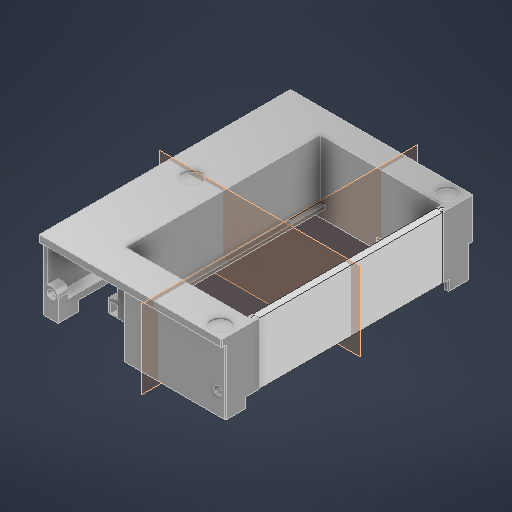
# Autodesk Inventor part: Kameraturm_Base_V3
Saved by Autodesk Inventor 2026.1 (Build 301233020, 233B)
## iProperties
Created: 2025-08-17
Part Number: Kameraturm_Base_V3
Material: Generic
Document SubType Name: Modeling
Designer: peter
Density: 1 g/cm^3
Appearance: Default
Author: peter
Autodesk Inventor part; units mm, degrees
sketch "Sketch1" plane through (0, 0, 0) normal (0, 0, 1) x (1, 0, 0)
  line L0 (135, 183) -> (0, 183) projected
  line L1 (0, 180) -> (0, 183) projected
  line L2 (0, 180) -> (135, 180) projected
  line L3 (135, 180) -> (135, 183) projected
  line L4 (0, -3) -> (135, -3) projected
  line L5 (135, 0) -> (135, -3) projected
  line L6 (135, 0) -> (0, 0) projected
  line L7 (0, 0) -> (0, -3) projected
  line L8 (0, 183) -> (135, 183)
  line L9 (135, 183) -> (135, -3)
  line L10 (135, -3) -> (0, -3)
  line L11 (0, -3) -> (0, 183)
  point P0 (135, 180)
  constraints: 8 end point, 2 parallel, 1 horizontal, 1 perpendicular
extrude "Extrusion1" add sketch "Sketch1" against normal blind 40 contours L9 L6 L11 L2
sketch "Sketch2" plane through (0, 0, 0) normal (0, 0, 1) x (1, 0, 0)
  line L0 (135, 180) -> (135, 0) construction
  line L1 (135, 90) -> (0, 90) construction
  line L2 (0, 0) -> (0, 180) construction
  line L3 (40, 165) -> (130, 165)
  line L4 (130, 165) -> (130, 15)
  line L5 (130, 15) -> (40, 15)
  line L6 (40, 15) -> (40, 165)
  line L7 (40, 165) -> (130, 15) construction
  line L8 (130, 165) -> (40, 15) construction
  line L9 (40, 15) -> (130, 15)
  line L10 (130, 15) -> (130, 21)
  line L11 (130, 21) -> (40, 21)
  line L12 (40, 21) -> (40, 15)
  point P0 (85, 90)
  dimension "d2" = 90
  dimension "d3" = 150
  dimension "d4" = 5
  dimension "d67" = 6
  constraints: 22 end point, 4 midpoint, 4 parallel, 2 horizontal, 2 perpendicular, 2 point on line
  measures "d2" distance of L4.end L5.end
  measures "d3" distance of L3.end L4.end
  measures "d4" distance between parallel lines of L0 L4
  measures "d67" distance of L10.end L9.end
extrude "Extrusion2" cut sketch "Sketch2" against normal through all contours L3 L4 L11 L6
sketch "Sketch3" plane through (0, 0, 0) normal (0, 0, 1) x (1, 0, 0)
  line L0 (135, 0) -> (0, 0) projected
  line L1 (60, 0) -> (3, 0)
  line L2 (3, 0) -> (3, 18)
  line L3 (3, 18) -> (60, 18)
  line L4 (60, 18) -> (60, 0)
  line L5 (3, 18) -> (37, 18)
  line L6 (37, 18) -> (37, 40.7573)
  line L7 (37, 40.7573) -> (3, 40.7573)
  line L8 (3, 40.7573) -> (3, 18)
  line L9 (40, 21) -> (40, 165) projected
  line L10 (0, 180) -> (0, 0) projected
  line L11 (130, 21) -> (40, 21) projected
  point P0 (37, 18)
  dimension "d8" = 3
  dimension "d9" = 3
  dimension "d10" = 60
  dimension "d68" = 3
  constraints: 16 end point, 4 parallel, 2 horizontal, 2 perpendicular, 1 point on line
  measures "d8" distance between parallel lines of L9 L6
  measures "d9" distance between parallel lines of L10 L8
  measures "d10" distance between parallel lines of L10 L4
  measures "d68" distance between parallel lines of L11 L3
extrude "Extrusion3" cut sketch "Sketch3" against normal blind 36
ref_plane "Work Plane1" through (-62, 12.5, -48) normal (0, 0, 1) x (1, 0, 0)
sketch "Sketch4" plane through (0, 0, -40) normal (0, 0, -1) x (-1, 0, 0)
  line L0 (0, -2.5) -> (0, 22) projected
  line L1 (0, 158) -> (0, 182.5) projected
  line L2 (125, -2.5) -> (125, 182.5) projected
  line L3 (-478, 162.5) -> (92, 162.5) projected
  line L4 (92, 17.5) -> (-478, 17.5) projected
  line L5 (-135, 180) -> (-135, 0) projected
  line L6 (0, 0) -> (-135, 0)
  line L7 (-135, 0) -> (-135, 15)
  line L8 (-135, 15) -> (0, 15)
  line L9 (0, 15) -> (0, 0)
  line L10 (0, 180) -> (-135, 180) projected
  line L11 (0, 180) -> (-135, 180)
  line L12 (-135, 180) -> (-135, 165)
  line L13 (-135, 165) -> (0, 165)
  line L14 (0, 165) -> (0, 180)
  line L15 (125, 182.5) -> (0, 182.5) projected
  line L16 (0, -2.5) -> (125, -2.5) projected
  line L17 (100, 22) -> (0, 22) projected
  line L18 (100, 22) -> (100, 158) projected
  line L19 (0, 158) -> (100, 158) projected
  circle A0 centre (80, 170.25) radius 7.05 projected
  circle A1 centre (40, 170.25) radius 7.05 projected
  point P0 (100, 22.5)
  point P1 (100, 157.5)
  point P2 (-130, 15)
  point P3 (-130, 165)
  constraints: 16 end point, 4 parallel, 2 horizontal, 2 horizontal alignment, 2 perpendicular, 2 point on line
extrude "Extrusion4" add sketch "Sketch4" along normal up to surface (8 mm away) contours L6 L5 L8 L0 | L1 L13 L5 L10
sketch "Sketch5" plane through (0, 180, 0) normal (0, 1, 0) x (1, 0, 0)
  line L0 (135, 25) -> (0, 25) projected
  line L1 (60, 0) -> (135, 0) projected
  line L2 (135, 0) -> (0, 0)
  line L3 (0, 0) -> (0, 25)
  line L4 (0, 25) -> (135, 25)
  line L5 (135, 25) -> (135, 0)
  point P0 (0, 0)
  constraints: 8 end point, 2 parallel, 1 horizontal, 1 perpendicular
ref_plane "Work Plane2" through (-120, 183, -97.3) normal (0, 1, 0) x (0, 0, 1)
extrude "Extrusion5" add sketch "Sketch5" along normal up to surface (3 mm away)
sketch "Sketch8" plane through (0, 0, 0) normal (0, 0, 1) x (1, 0, 0)
  line L0 (670, 183) -> (135, 183) projected
  line L1 (0, -3) -> (135, -3) projected
  line L2 (135, 183) -> (0, 183)
  line L3 (0, 183) -> (0, -3)
  line L4 (0, -3) -> (135, -3)
  line L5 (135, -3) -> (135, 183)
  line L6 (3, 0) -> (3, 40.7573) projected
  line L7 (3, 40.7573) -> (37, 40.7573) projected
  line L8 (37, 40.7573) -> (37, 18) projected
  line L9 (37, 18) -> (60, 18) projected
  line L10 (60, 18) -> (60, 0) projected
  line L11 (60, 0) -> (135, 0) projected
  line L12 (135, 0) -> (135, 183) projected
  line L13 (135, 183) -> (0, 183) projected
  line L14 (0, 183) -> (0, 0) projected
  line L15 (0, 0) -> (3, 0) projected
  line L16 (130, 165) -> (130, 21) projected
  line L17 (40, 21) -> (40, 165) projected
  line L18 (40, 165) -> (130, 165) projected
  line L19 (60, 0) -> (0, 0)
  line L20 (130, 21) -> (40, 21) projected
  constraints: 10 end point, 3 parallel, 1 horizontal, 1 perpendicular
extrude "Extrusion8" add sketch "Sketch8" along normal blind 5
sketch "Sketch9" plane through (0, 0, 5) normal (0, 0, 1) x (1, 0, 0)
  circle A0 centre (125, 174) radius 7.05
  circle A1 centre (125, 6) radius 7.05
  line L0 (135, -3) -> (135, 183) projected
  line L1 (135, 183) -> (0, 183) projected
  line L2 (0, -3) -> (135, -3) projected
  line L3 (0, 183) -> (0, -3) projected
  circle A2 centre (20, 90) radius 7.05
  line L4 (0, 90) -> (40, 90) construction
  line L5 (40, 165) -> (40, 21) projected
  point P0 (0, 0)
  point P1 (40, 15)
  dimension "d31" = 14.1
  dimension "d35" = 10
  dimension "d36" = 9
  dimension "d37" = 9
  constraints: 3 centre point, 3 midpoint, 2 end point, 2 equal radius, 1 coincident, 1 horizontal alignment, 1 point on line, 1 vertical alignment
  measures "d31" diameter of A0
  measures "d35" distance from line of L0 A0.centre
  measures "d36" distance from line of L1 A0.centre
  measures "d37" distance from line of L2 A1.centre
extrude "Extrusion9" cut sketch "Sketch9" against normal blind 1.5 contours A0 | A1 | A2
chamfer "Chamfer1" distance 0.5 angle 45 14 edges at (135, 183, 2.5) (135, 183, -12.5) (0, 183, -12.5) (0, 183, 2.5) (0, 0, -24) (135, 0, -24) (135, -3, 2.5) (0, -3, 2.5) (135, 180, -36.5) (0, 180, -36.5) (135, 15, -44) (135, 165, -44) (0, 15, -44) (0, 165, -44)
ref_plane "Work Plane3" through (0, 0, 0) normal (0, 0, 1) x (1, 0, 0)
ref_plane "Work Plane4" through (0, 0, -3) normal (0, 0, -1) x (-1, 0, 0)
sketch "Sketch12" plane through (0.5, 180, -25) normal (0, 1, 0) x (1, 0, 0)
  arc A0 (107.5, 4.5) -> (107.5, 9.5) centre (107.5, 7) ccw projected
  arc A1 (106.5, 9.5) -> (106.5, 4.5) centre (106.5, 7) ccw projected
  arc A2 (26.5, 9.5) -> (26.5, 4.5) centre (26.5, 7) ccw projected
  arc A3 (27.5, 4.5) -> (27.5, 9.5) centre (27.5, 7) ccw projected
  line L0 (107.5, 7) -> (106.5, 7)
  line L1 (27.5, 7) -> (26.5, 7)
  circle A4 centre (107, 7) radius 3.2
  circle A5 centre (27, 7) radius 3.2
  point P0 (-0.5, -25)
  dimension "d53" = 6.4
  dimension "d54" = 6.4
  constraints: 4 end point, 2 centre point, 2 horizontal, 2 midpoint
  measures "d53" diameter of A4
  measures "d54" diameter of A5
extrude "Extrusion12" cut sketch "Sketch12" against normal blind 12
sketch "Sketch13" plane through (3, 0, -36) normal (0, -1, 0) x (1, 0, 0)
  circle A0 centre (3, 4) radius 2.5 projected
  circle A1 centre (3, 4) radius 5
  line L0 (57, 0) -> (0, 0) projected
  line L1 (0, 0) -> (0, 36) projected
  line L2 (8, 4) -> (8, 0)
  line L3 (3, 9) -> (0, 9)
  circle A2 centre (3, 4) radius 3.2
  point P0 (-3, 36)
  dimension "d57" = 10
  dimension "d58" = 6.4
  constraints: 4 end point, 2 centre point, 2 coincident, 2 perpendicular, 2 point on circle, 2 point on line, 2 tangent
  measures "d57" diameter of A1
  measures "d58" diameter of A2
extrude "Extrusion13" add sketch "Sketch13" against normal blind 8 contours A1 L0 L1 A2 | L2 L0 A1 | A1 L1 L3 | A2 L1 picked at (0.1667, 4)
sketch "Sketch14" plane through (60, 0, -36) normal (0, -1, 0) x (1, 0, 0)
  circle A0 centre (-54, 4) radius 2.5 projected
  circle A1 centre (69, 4) radius 2.5 projected
  circle A2 centre (-54, 4) radius 3.2
  circle A3 centre (69, 4) radius 3.2
  point P0 (-60, 36)
  dimension "d61" = 6.4
  dimension "d62" = 6.4
  constraints: 2 centre point, 2 coincident
  measures "d61" diameter of A2
  measures "d62" diameter of A3
extrude "Extrusion14" cut sketch "Sketch14" against normal blind 12 contours A0 | A1 | A2 | A3
sketch "Sketch15" plane through (0, 0, -36) normal (0, 0, 1) x (1, 0, 0)
  line L0 (11, 8) -> (11, 0) projected
  line L1 (60, 0) -> (11, 0) projected
  line L2 (60, 18) -> (60, 0) projected
  line L3 (37, 18) -> (60, 18) projected
  line L4 (37, 40.7573) -> (37, 18) projected
  line L5 (3, 40.7573) -> (37, 40.7573) projected
  line L6 (3, 8) -> (3, 40.7573) projected
  line L7 (3, 8) -> (11, 8) projected
  line L8 (11, 0) -> (60, 0)
  line L9 (60, 0) -> (60, 18)
  line L10 (60, 18) -> (11, 18)
  line L11 (11, 18) -> (11, 0)
  line L12 (11, 18) -> (37, 18)
  line L13 (37, 18) -> (37, 40.7573)
  line L14 (37, 40.7573) -> (11, 40.7573)
  line L15 (11, 40.7573) -> (11, 18)
  point P0 (0, 0)
  constraints: 16 end point, 4 parallel, 2 horizontal, 2 perpendicular
extrude "Extrusion15" cut sketch "Sketch15" against normal through all contours L11 L10 L3 L2 L1 L0 | L15 L5 L4 L10
ref_plane "Work Plane5" through (0, 0, -40) normal (0, 0, -1) x (-1, 0, 0)
sketch "Sketch16" plane through (0, 0, -40) normal (0, 0, -1) x (-1, 0, 0)
  line L0 (-11, 40.7573) -> (-11, 15) projected
  line L1 (-11, 15) -> (-0.5, 15) projected
  line L2 (0, 14.5) -> (-0.5, 15) projected
  line L3 (0, 14.5) -> (0, 165.5) projected
  line L4 (-0.5, 165) -> (0, 165.5) projected
  line L5 (-0.5, 165) -> (-40, 165) projected
  line L6 (-40, 165) -> (-40, 21) projected
  line L7 (-40, 21) -> (-130, 21) projected
  line L8 (-130, 21) -> (-130, 165) projected
  line L9 (-130, 165) -> (-134.5, 165) projected
  line L10 (-135, 165.5) -> (-134.5, 165) projected
  line L11 (-135, 165.5) -> (-135, 14.5) projected
  line L12 (-134.5, 15) -> (-135, 14.5) projected
  line L13 (-134.5, 15) -> (-60, 15) projected
  line L14 (-60, 15) -> (-60, 18) projected
  line L15 (-60, 18) -> (-37, 18) projected
  line L16 (-37, 18) -> (-37, 40.7573) projected
  line L17 (-37, 40.7573) -> (-11, 40.7573) projected
  line L18 (-40, 21) -> (-130, 21)
  line L19 (-130, 21) -> (-130, 24)
  line L20 (-130, 24) -> (-40, 24)
  line L21 (-40, 24) -> (-40, 21)
  line L22 (-40, 21) -> (-43, 21)
  line L23 (-43, 21) -> (-43, 41)
  line L24 (-43, 41) -> (-40, 41)
  line L25 (-40, 41) -> (-40, 21)
  line L26 (-40, 41) -> (-43, 41)
  line L27 (-43, 41) -> (-43, 141)
  line L28 (-43, 141) -> (-40, 141)
  line L29 (-40, 141) -> (-40, 41)
  line L30 (-134.5, 165) -> (-0.5, 165) projected
  line L31 (-40, 141) -> (-43, 141)
  line L32 (-43, 141) -> (-43, 165)
  line L33 (-43, 165) -> (-40, 165)
  line L34 (-40, 165) -> (-40, 141)
  point P0 (0, 0)
  point P1 (-43, 24)
  point P2 (-43, 41)
  dimension "d72" = 3
  dimension "d73" = 3
  dimension "d74" = 20
  dimension "d75" = 3
  dimension "d76" = 100
  dimension "d77" = 3
  constraints: 32 end point, 8 parallel, 4 horizontal, 4 perpendicular, 1 point on line, 1 vertical alignment
  measures "d72" distance of L18.end L19.end
  measures "d73" distance of L23.end L24.end
  measures "d74" distance of L22.end L23.end
  measures "d75" distance of L27.end L28.end
  measures "d76" distance of L26.end L27.end
  measures "d77" distance of L32.end L33.end
extrude "Extrusion16" add sketch "Sketch16" against normal blind 2 separate body contours L6 L28 L32 L30 | L6 L20 L23 L24 | L6 L7 L23 L20 | L20 L23 L7 L8
extrude "Extrusion17" add sketch "Sketch16" against normal blind 2 contours L17 L16 L15 L14 L13 L12 L11 L10 L9 L8 L7 L6 L5 L4 L3 L2 L1 L0 | L6 L24 L27 L28 bodies 1
sketch "Sketch17" plane through (0, 0, -40) normal (0, 0, -1) x (-1, 0, 0)
  line L0 (-134.5, 165) -> (-135, 165.5) construction
  line L1 (-135, 14.5) -> (-135, 165.5) construction
  line L2 (-135, 0.5) -> (-135, 14.5) construction
  line L3 (-134.5, 0) -> (-135, 0.5) construction
  line L4 (-60, 0) -> (-134.5, 0) construction
  line L5 (-60, 15) -> (-60, 0) construction
  line L6 (-134.5, 15) -> (-60, 15) construction
  line L7 (-135, 14.5) -> (-134.5, 15) construction
  line L8 (-130, 165) -> (-134.5, 165) construction
  line L9 (-130, 165) -> (-130, 21) construction
  line L10 (-130, 21) -> (-40, 21) construction
  line L11 (-40, 21) -> (-40, 41) construction
  line L12 (-40, 41) -> (-43, 41) construction
  line L13 (-43, 41) -> (-43, 141) construction
  line L14 (-43, 141) -> (-40, 141) construction
  line L15 (-40, 141) -> (-40, 165) construction
  line L16 (-0.5, 165) -> (-40, 165) construction
  line L17 (0, 165.5) -> (-0.5, 165) construction
  line L18 (0, 179.5) -> (0, 165.5) construction
  line L19 (-0.5, 180) -> (0, 179.5) construction
  line L20 (-134.5, 180) -> (-0.5, 180) construction
  line L21 (-135, 179.5) -> (-134.5, 180) construction
  line L22 (-135, 165.5) -> (-135, 179.5) construction
  line L23 (-60, 18) -> (-60, 15) construction
  line L24 (-37, 18) -> (-60, 18) construction
  line L25 (-37, 40.7573) -> (-37, 18) construction
  line L26 (-11, 40.7573) -> (-37, 40.7573) construction
  line L27 (-11, 15) -> (-11, 40.7573) construction
  line L28 (-11, 0) -> (-11, 15) construction
  line L29 (-0.5, 0) -> (-11, 0) construction
  line L30 (0, 0.5) -> (-0.5, 0) construction
  line L31 (0, 14.5) -> (0, 0.5) construction
  line L32 (0, 165.5) -> (0, 14.5) construction
  line L33 (-40, 165) -> (-130, 165) construction
  line L34 (-11, 15) -> (-0.5, 15) construction
  line L35 (-0.5, 15) -> (0, 14.5) construction
  line L36 (-40, 165) -> (-40, 141) construction
  line L37 (-40, 141) -> (-43, 141) construction
  line L38 (-43, 141) -> (-43, 165) construction
  line L39 (-43, 165) -> (-40, 165) construction
  line L40 (-130, 24) -> (-43, 24) construction
  line L41 (-43, 24) -> (-43, 41) construction
  line L42 (-43, 41) -> (-40, 41) construction
  line L43 (-40, 41) -> (-40, 21) construction
  line L44 (-40, 21) -> (-130, 21) construction
  line L45 (-130, 21) -> (-130, 24) construction
  line L46 (-130, 24) -> (-43, 24)
  line L47 (-43, 24) -> (-43, 165)
  line L48 (-43, 165) -> (-130, 165)
  line L49 (-130, 165) -> (-130, 24)
  line L50 (-130, 25) -> (-44, 25)
  line L51 (-44, 25) -> (-44, 165)
  line L52 (-44, 165) -> (-130, 165)
  line L53 (-130, 165) -> (-130, 25)
  point P0 (0, 0)
  dimension "d82" = 1
  dimension "d83" = 1
  constraints: 16 end point, 4 parallel, 2 horizontal, 2 perpendicular, 2 point on line
  measures "d82" distance between parallel lines of L13 L51
  measures "d83" distance between parallel lines of L50 L40
extrude "Extrusion18" add sketch "Sketch17" against normal blind 2 contours L49 L50 L51 L48 L47 L46 bodies 1
sketch "Sketch18" plane through (0, 0, -40) normal (0, 0, -1) x (-1, 0, 0)
  line L0 (-43, 41) -> (-43, 24) projected
  line L1 (-43, 24) -> (-130, 24) projected
  line L2 (-130, 24) -> (-130, 21) projected
  line L3 (-130, 21) -> (-40, 21) projected
  line L4 (-40, 21) -> (-40, 41) projected
  line L5 (-40, 41) -> (-43, 41) projected
  line L6 (-134.5, 165) -> (-135, 165.5) projected
  line L7 (-135, 14.5) -> (-135, 165.5) projected
  line L8 (-135, 0.5) -> (-135, 14.5) projected
  line L9 (-134.5, 0) -> (-135, 0.5) projected
  line L10 (-60, 0) -> (-134.5, 0) projected
  line L11 (-60, 15) -> (-60, 0) projected
  line L12 (-134.5, 15) -> (-60, 15) projected
  line L13 (-135, 14.5) -> (-134.5, 15) projected
  line L14 (-130, 165) -> (-134.5, 165) projected
  line L15 (-130, 165) -> (-130, 25) projected
  line L16 (-130, 25) -> (-44, 25) projected
  line L17 (-44, 25) -> (-44, 165) projected
  line L18 (-43, 165) -> (-44, 165) projected
  line L19 (-43, 165) -> (-43, 141) projected
  line L20 (-43, 141) -> (-40, 141) projected
  line L21 (-40, 141) -> (-40, 165) projected
  line L22 (-0.5, 165) -> (-40, 165) projected
  line L23 (0, 165.5) -> (-0.5, 165) projected
  line L24 (0, 179.5) -> (0, 165.5) projected
  line L25 (-0.5, 180) -> (0, 179.5) projected
  line L26 (-134.5, 180) -> (-0.5, 180) projected
  line L27 (-135, 179.5) -> (-134.5, 180) projected
  line L28 (-135, 165.5) -> (-135, 179.5) projected
  line L29 (-60, 18) -> (-60, 15) projected
  line L30 (-37, 18) -> (-60, 18) projected
  line L31 (-37, 40.7573) -> (-37, 18) projected
  line L32 (-11, 40.7573) -> (-37, 40.7573) projected
  line L33 (-11, 15) -> (-11, 40.7573) projected
  line L34 (-11, 15) -> (-0.5, 15) projected
  line L35 (-0.5, 15) -> (0, 14.5) projected
  line L36 (0, 165.5) -> (0, 14.5) projected
  line L37 (-44, 165) -> (-130, 165) projected
  line L38 (-40, 165) -> (-43, 165) projected
  line L39 (-11, 0) -> (-11, 15) projected
  line L40 (-0.5, 0) -> (-11, 0) projected
  line L41 (0, 0.5) -> (-0.5, 0) projected
  line L42 (0, 14.5) -> (0, 0.5) projected
  line L43 (-40, 165) -> (-40, 141) projected
  line L44 (-40, 141) -> (-43, 141) projected
  line L45 (-43, 141) -> (-43, 165) projected
  line L46 (-43, 165) -> (-40, 165) projected
  line L47 (-130, 24) -> (-43, 24) projected
  line L48 (-43, 24) -> (-43, 41) projected
  line L49 (-43, 41) -> (-40, 41) projected
  line L50 (-40, 41) -> (-40, 21) projected
  line L51 (-40, 21) -> (-130, 21) projected
  line L52 (-130, 21) -> (-130, 24) projected
  point P0 (0, 0)
extrude "Extrusion19" add sketch "Sketch18" along normal blind 0.6 contours L5 L4 L3 L2 L1 L0 | L14 L15 L16 L17 L18 L19 L20 L21 L22 L23 L36 L35 L34 L33 L32 L31 L30 L29 L12 L13 L7 L6 | L38 L21 L20 L19 bodies 1
sketch "Sketch19" plane through (60, 0, -48) normal (0, 0, -1) x (-1, 0, 0)
  line L0 (0, 15) -> (-74.5, 15) projected
  line L1 (-22, 15) -> (-72, 15)
  line L2 (-72, 15) -> (-72, 2)
  line L3 (-72, 2) -> (-22, 2)
  line L4 (-22, 2) -> (-22, 15)
  line L5 (16, 165) -> (16, 25) projected
  line L6 (-74.5, 165) -> (59.5, 165) projected
  line L7 (-72, 165) -> (-22, 165)
  line L8 (-22, 165) -> (-22, 178)
  line L9 (-22, 178) -> (-72, 178)
  line L10 (-72, 178) -> (-72, 165)
  point P0 (60, 0)
  dimension "d89" = 38
  dimension "d92" = 50
  dimension "d93" = 13
  dimension "d94" = 13
  constraints: 16 end point, 5 parallel, 2 horizontal, 2 perpendicular, 2 point on line, 1 vertical alignment
  measures "d89" distance from line of L5 L1.start
  measures "d92" distance of L2.end L3.end
  measures "d93" distance of L3.end L1.start
  measures "d94" distance between parallel lines of L6 L9
extrude "Extrusion20" cut sketch "Sketch19" against normal blind 8.5 bodies 1
sketch "Sketch20" plane through (60, 0, -39.5) normal (0, 0, -1) x (-1, 0, 0)
  line L0 (-4.8389, 5.5) -> (-96.0854, 5.5) construction
  line L1 (-4.8389, 174.5) -> (-96.0854, 174.5) construction
  line L2 (-22, 2) -> (-72, 2) construction
  line L3 (-72, 178) -> (-22, 178) construction
  point P0 (60, 0)
  point P1 (-26.5, 5.5)
  point P2 (-42, 5.5)
  point P3 (-57.5, 5.5)
  point P4 (-47, 2)
  point P5 (-57.5, 174.5)
  point P6 (-42, 174.5)
  point P7 (-26.5, 174.5)
  point P8 (-47, 2)
  dimension "d97" = 3.5
  dimension "d98" = 3.5
  dimension "d99" = 15.5
  dimension "d100" = 15.5
  dimension "d149" = 5
  constraints: 6 point on line, 4 end point, 3 vertical alignment, 2 horizontal, 2 midpoint
  measures "d97" distance between parallel lines of L2 L0
  measures "d98" distance between parallel lines of L3 L1
  measures "d99" distance of point (-42, 5.5) point (-26.5, 5.5)
  measures "d100" distance of point (-42, 5.5) point (-57.5, 5.5)
  measures "d149" horizontal distance of point (-47, 2) point (-42, 5.5)
hole "Hole1" at (102, 5.5, -39.5) at (117.5, 5.5, -39.5) at (117.5, 174.5, -39.5) at (102, 174.5, -39.5) direction (0, 0, 1) diameter 4 depth 6 bodies 1
sketch "Sketch21" plane through (82, 2, -48) normal (1, 0, 0) x (0, 0, -1)
  circle A0 centre (-3.7, 6.5) radius 2.5
  line L0 (-7.4, 13) -> (0, 13) projected
  line L1 (0, 13) -> (0, 0) projected
  line L2 (-1.2, 9) -> (-6.2, 9)
  line L3 (-6.2, 9) -> (-6.2, 4)
  line L4 (-6.2, 4) -> (-1.2, 4)
  line L5 (-1.2, 4) -> (-1.2, 9)
  line L6 (-1.2, 9) -> (-6.2, 4) construction
  line L7 (-6.2, 9) -> (-1.2, 4) construction
  point P0 (-48, -2)
  point P1 (-3.7, 13)
  point P2 (0, 6.5)
  point P3 (-1.2, 6.5)
  point P4 (-3.7, 4)
  point P5 (-3.7, 9)
  point P6 (-6.2, 6.5)
  dimension "d112" = 5
  dimension "d147" = 5
  dimension "d148" = 5
  constraints: 12 end point, 4 midpoint, 2 parallel, 1 centre point, 1 horizontal, 1 horizontal alignment, 1 perpendicular, 1 vertical alignment
  measures "d112" diameter of A0
  measures "d147" distance of L4.end L3.end
  measures "d148" distance of L3.end L2.end
extrude "Extrusion22" cut sketch "Sketch21" against normal blind 30.75 bodies 1
sketch "Sketch22" plane through (0, 0, -40.6) normal (0, 0, -1) x (-1, 0, 0)
  line L0 (-37, 40.7573) -> (-11, 40.7573) projected
  line L1 (-82, 165) -> (-0.5, 165) projected
  line L2 (-32, 40.7573) -> (-37, 40.7573)
  line L3 (-37, 40.7573) -> (-37, 165)
  line L4 (-37, 165) -> (-32, 165)
  line L5 (-32, 165) -> (-32, 40.7573)
  line L6 (-44, 165) -> (-44, 25) projected
  line L7 (-32, 165) -> (-37, 165)
  line L8 (-37, 165) -> (-37, 173)
  line L9 (-37, 173) -> (-32, 173)
  line L10 (-32, 173) -> (-32, 165)
  line L11 (-40, 21) -> (-40, 165) projected
  point P0 (0, 0)
  dimension "d115" = 5
  dimension "d119" = 5
  dimension "d120" = 8
  dimension "d121" = 3
  constraints: 16 end point, 4 parallel, 2 horizontal, 2 perpendicular, 2 point on line
  measures "d115" distance of L3.end L4.end
  measures "d119" distance of L8.end L9.end
  measures "d120" distance of L7.end L8.end
  measures "d121" distance between parallel lines of L3 L11
extrude "Extrusion23" cut sketch "Sketch22" against normal blind 8 bodies 1
sketch "Sketch23" plane through (32, 173, -40.6) normal (0, -1, 0) x (1, 0, 0)
  line L0 (0, 0) -> (5, 0) projected
  line L1 (5, 0) -> (5, 8) projected
  line L2 (5, 8) -> (0, 8) projected
  line L3 (0, 0) -> (0, 8) projected
  line L4 (5, 8) -> (50, -0.9)
  line L5 (50, -7.4) -> (50, 1.1) projected
  line L6 (5, 0) -> (50, -5.9)
  point P0 (-32, 40.6)
  dimension "d122" = 5
  dimension "d123" = 1.5
  constraints: 4 end point, 2 point on line
  measures "d122" distance of L6.end L4.end
  measures "d123" distance of L5.start L6.end
extrude "Extrusion24" cut sketch "Sketch23" along normal blind 5 contours L1 L4 L5 L6 bodies 1
fillet "Fillet1" radius 5 1 edges at (37, 168, -36.6)
chamfer "Chamfer3" distance 5 angle 45 1 edges at (82, 173, -44)
fillet "Fillet2" radius 7 1 edges at (32, 173, -36.6)
sketch "Sketch24" plane through (0, 0, -40.6) normal (0, 0, -1) x (-1, 0, 0)
  line L0 (-32, 40.7573) -> (-37, 40.7573) projected
  line L1 (-44, 165) -> (-37.4174, 165) projected
  line L2 (-32, 40.7573) -> (-38.5033, 40.7573)
  line L3 (-38.5033, 40.7573) -> (-38.5033, 165)
  line L4 (-38.5033, 165) -> (-32, 165)
  line L5 (-32, 165) -> (-32, 40.7573)
  line L6 (-32, 165) -> (-38.5033, 165)
  line L7 (-38.5033, 165) -> (-38.5033, 166)
  line L8 (-38.5033, 166) -> (-32, 166)
  line L9 (-32, 166) -> (-32, 165)
  point P0 (0, 0)
  dimension "d133" = 1
  constraints: 16 end point, 4 parallel, 2 horizontal, 2 perpendicular, 1 point on line
  measures "d133" distance of L6.end L7.end
extrude "Extrusion25" add sketch "Sketch24" against normal blind 0.6 bodies 1
chamfer "Chamfer4" distance 1.05 distance2 0.6 1 edges at (35, 166, -40) measured on face at (35, 165.5, -40)
chamfer "Chamfer5" distance 1 angle 45 4 edges at (82, 8.5, -41.8) (82, 6, -44.3) (82, 11, -44.3) (82, 8.5, -46.8)
sketch "Sketch25" plane through (37, 18, 0) normal (0, -1, 0) x (1, 0, 0)
  line L0 (23, -40.6) -> (0, -40.6) projected
  line L1 (0, -40.6) -> (-6.5, -40.6)
  line L2 (-6.5, -40.6) -> (-6.5, -30.6)
  line L3 (-6.5, -30.6) -> (0, -30.6)
  line L4 (0, -30.6) -> (0, -40.6)
  line L5 (-5, -32.6) -> (0, -32.6) projected
  line L6 (-5, -40) -> (-5, -32.6) projected
  line L7 (-5, -40) -> (0, -40) projected
  point P0 (-37, 0)
  dimension "d140" = 2
  dimension "d141" = 1.5
  constraints: 8 end point, 2 parallel, 1 horizontal, 1 perpendicular
  measures "d140" distance between parallel lines of L3 L5
  measures "d141" distance between parallel lines of L2 L6
extrude "Extrusion26" add sketch "Sketch25" against normal up to surface (22.7573 mm away) contours L1 L2 L3 L4 L5 L6 L7 bodies 1
chamfer "Chamfer6" distance 1.5 distance2 6.5 1 edges at (37, 29.3786, -30.6) measured on face at (37, 29.3786, -30.1)
ref_plane "Work Plane6" through (40, 93, 5) normal (0, -1, 0) x (1, 0, 0)
ref_plane "Work Plane7" through (85, 21, 5) normal (1, 0, 0) x (0, 0, -1)
thicken "Verdickung2" operation add thickness 2 both sides no extend neighbours no toward (0, 0, -1) bodies 1 faces at (104.6667, 167.5, -39.5)
thicken "Verdickung3" operation add thickness 2 both sides no extend neighbours no toward (0, 0, -1) bodies 1 faces at (105.3333, 12.5, -39.5)
sketch "Skizze26" plane through (0, 0, 5) normal (0, 0, 1) x (1, 0, 0)
  line L0 (0.5, -3) -> (0, -2.5) projected
  line L1 (0.5, -3) -> (134.5, -3) projected
  line L2 (135, -2.5) -> (134.5, -3) projected
  line L3 (135, -2.5) -> (135, 182.5) projected
  line L4 (134.5, 183) -> (135, 182.5) projected
  line L5 (134.5, 183) -> (0.5, 183) projected
  line L6 (0, 182.5) -> (0.5, 183) projected
  line L7 (0, 182.5) -> (0, -2.5) projected
  circle A0 centre (125, 174) radius 7.05 projected
  circle A1 centre (125, 6) radius 7.05 projected
  circle A2 centre (20, 90) radius 7.05 projected
  line L8 (130, 165) -> (130, 21) projected
  line L9 (130, 21) -> (40, 21) projected
  line L10 (40, 21) -> (40, 165) projected
  line L11 (40, 165) -> (130, 165) projected
  line L12 (135, 165.5) -> (135, 14.5) projected
  line L13 (130, 21) -> (135, 21)
  line L14 (135, 21) -> (135, 165)
  line L15 (135, 165) -> (130, 165)
  line L16 (130, 165) -> (130, 21)
  line L17 (130, 25) -> (135, 25)
  line L18 (135, 25) -> (135, 161)
  line L19 (135, 161) -> (130, 161)
  line L20 (130, 161) -> (130, 25)
  line L21 (133.55, 28) -> (131.45, 28)
  line L22 (131.45, 28) -> (131.45, 22)
  line L23 (131.45, 22) -> (133.55, 22)
  line L24 (133.55, 22) -> (133.55, 28)
  line L25 (133.55, 28) -> (131.45, 22) construction
  line L26 (131.45, 28) -> (133.55, 22) construction
  line L27 (131.45, 158) -> (133.55, 158)
  line L28 (133.55, 158) -> (133.55, 164)
  line L29 (133.55, 164) -> (131.45, 164)
  line L30 (131.45, 164) -> (131.45, 158)
  line L31 (131.45, 158) -> (133.55, 164) construction
  line L32 (133.55, 158) -> (131.45, 164) construction
  point P0 (0, 0)
  point P1 (132.5, 21)
  point P2 (132.5, 25)
  point P3 (132.5, 165)
  point P4 (132.5, 161)
  point P5 (131.45, 161)
  point P6 (133.55, 161)
  point P7 (133.55, 25)
  point P8 (131.45, 25)
  dimension "d156" = 4
  dimension "d157" = 4
  dimension "d158" = 2.1
  dimension "d159" = 6
  dimension "d160" = 2.1
  dimension "d161" = 6
  constraints: 40 end point, 8 midpoint, 8 parallel, 4 horizontal, 4 perpendicular, 3 point on line, 1 coincident
  measures "d156" distance of point (132.5, 21) point (132.5, 25)
  measures "d157" distance of point (132.5, 165) point (132.5, 161)
  measures "d158" distance of L23.end L22.end
  measures "d159" distance of L22.end L21.end
  measures "d160" distance of L29.end L28.end
  measures "d161" distance of L28.end L27.end
extrude "Extrusion27" cut sketch "Skizze26" against normal through all contours L17 L24 L21 L22 L8 L19 L30 L27 L28 L3 | L17 L22 L21 L24 | L28 L27 L30 L19 bodies 1
extrude "Extrusion28" cut sketch "Skizze26" against normal blind 42.5 contours L24 L23 L22 L17 | L19 L30 L29 L28 bodies 1
sketch "Skizze27" plane through (0, 0, 5) normal (0, 0, 1) x (1, 0, 0)
  circle A0 centre (20, 90) radius 7.05 projected
  circle A1 centre (125, 6) radius 7.05 projected
  circle A2 centre (125, 174) radius 7.05 projected
  line L0 (131.45, 161) -> (131.45, 164) projected
  line L1 (131.45, 164) -> (133.55, 164) projected
  line L2 (133.55, 164) -> (133.55, 161) projected
  line L3 (133.55, 161) -> (135, 161) projected
  line L4 (135, 161) -> (135, 182.5) projected
  line L5 (134.5, 183) -> (135, 182.5) projected
  line L6 (134.5, 183) -> (0.5, 183) projected
  line L7 (0, 182.5) -> (0.5, 183) projected
  line L8 (0, 182.5) -> (0, -2.5) projected
  line L9 (0.5, -3) -> (0, -2.5) projected
  line L10 (0.5, -3) -> (134.5, -3) projected
  line L11 (135, -2.5) -> (134.5, -3) projected
  line L12 (135, -2.5) -> (135, 25) projected
  line L13 (135, 25) -> (133.55, 25) projected
  line L14 (133.55, 25) -> (133.55, 22) projected
  line L15 (133.55, 22) -> (131.45, 22) projected
  line L16 (131.45, 22) -> (131.45, 25) projected
  line L17 (131.45, 25) -> (130, 25) projected
  line L18 (130, 25) -> (130, 21) projected
  line L19 (130, 21) -> (40, 21) projected
  line L20 (40, 21) -> (40, 165) projected
  line L21 (40, 165) -> (130, 165) projected
  line L22 (130, 165) -> (130, 161) projected
  line L23 (130, 161) -> (131.45, 161) projected
  line L24 (130, 25) -> (135, 25) construction
  line L25 (135, 25) -> (135, 161) construction
  line L26 (135, 161) -> (130, 161) construction
  line L27 (130, 161) -> (130, 25) construction
  line L28 (133.5, 27.9) -> (131.5, 27.9)
  line L29 (131.5, 27.9) -> (131.5, 22.1)
  line L30 (131.5, 22.1) -> (133.5, 22.1)
  line L31 (133.5, 22.1) -> (133.5, 27.9)
  line L32 (133.5, 27.9) -> (131.5, 22.1) construction
  line L33 (131.5, 27.9) -> (133.5, 22.1) construction
  line L34 (133.5, 163.9) -> (131.5, 163.9)
  line L35 (131.5, 163.9) -> (131.5, 158.1)
  line L36 (131.5, 158.1) -> (133.5, 158.1)
  line L37 (133.5, 158.1) -> (133.5, 163.9)
  line L38 (133.5, 163.9) -> (131.5, 158.1) construction
  line L39 (131.5, 163.9) -> (133.5, 158.1) construction
  line L40 (135, 93) -> (130, 93) construction
  line L41 (135, 160.9) -> (130, 160.9)
  line L42 (130, 160.9) -> (130, 25.1)
  line L43 (130, 25.1) -> (135, 25.1)
  line L44 (135, 25.1) -> (135, 160.9)
  line L45 (135, 160.9) -> (130, 25.1) construction
  line L46 (130, 160.9) -> (135, 25.1) construction
  point P0 (0, 0)
  point P1 (132.5, 25)
  point P2 (132.5, 161)
  point P3 (132.5, 93)
  point P4 (133.5, 25.1)
  point P5 (133.5, 160.9)
  point P6 (131.5, 160.9)
  point P7 (131.5, 25.1)
  dimension "d164" = 2
  dimension "d165" = 5.8
  dimension "d166" = 2
  dimension "d167" = 5.8
  dimension "d168" = 0.1
  constraints: 46 end point, 11 midpoint, 8 parallel, 4 horizontal, 4 perpendicular, 1 vertical alignment
  measures "d164" distance of L30.end L29.end
  measures "d165" distance of L29.end L28.end
  measures "d166" distance of L36.end L35.end
  measures "d167" distance of L35.end L34.end
  measures "d168" distance between parallel lines of L24 L43
extrude "Extrusion29" add sketch "Skizze27" against normal blind 42.4 separate body contours L31 L43 L29 L28 | L28 L29 L43 L42 L41 L35 L36 L37 L44 L31 | L31 L30 L29 L43 | L41 L35 L34 L37 | L37 L36 L35 L41
sketch "Skizze28" plane through (0, 0, -37.4) normal (0, 0, -1) x (-1, 0, 0)
  line L0 (-133.5, 25.1) -> (-133.5, 22.1) projected
  line L1 (-133.5, 22.1) -> (-131.5, 22.1) projected
  line L2 (-131.5, 22.1) -> (-131.5, 25.1) projected
  line L3 (-131.5, 25.1) -> (-130, 25.1) projected
  line L4 (-130, 25.1) -> (-130, 160.9) projected
  line L5 (-130, 160.9) -> (-131.5, 160.9) projected
  line L6 (-131.5, 160.9) -> (-131.5, 163.9) projected
  line L7 (-131.5, 163.9) -> (-133.5, 163.9) projected
  line L8 (-133.5, 163.9) -> (-133.5, 160.9) projected
  line L9 (-133.5, 160.9) -> (-135, 160.9) projected
  line L10 (-135, 160.9) -> (-135, 25.1) projected
  line L11 (-135, 25.1) -> (-133.5, 25.1) projected
  line L12 (-135, 25.1) -> (-130, 25.1)
  line L13 (-130, 25.1) -> (-130, 160.9)
  line L14 (-130, 160.9) -> (-135, 160.9)
  line L15 (-135, 160.9) -> (-135, 25.1)
  point P0 (0, 0)
  constraints: 8 end point, 2 parallel, 1 horizontal, 1 perpendicular
extrude "Extrusion30" add sketch "Skizze28" along normal up to surface (3.2 mm away) contours L11 L10 L9 L14 L5 L4 L3 L12 bodies 3
body "Solid1"
body "Solid2"
